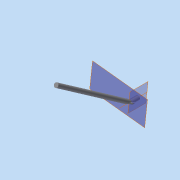
# Autodesk Inventor part: cellSTORM_lightpath
Saved by Autodesk Inventor 2019.4 (Build 234330000, 330)
## iProperties
Created: 2020-04-25
Part Number: cellSTORM_lightpath
Material: Generic
Document SubType Name: Modeling
Designer: diederichbenedict
Density: 1 g/cm^3
Appearance: Default
Mass: 3.01644 g
Surface Area: 25.0036 cm^2
Volume: 3.01644 cm^3
Author: diederichbenedict
Autodesk Inventor part; units mm, degrees
ref_plane "YZ Plane" through (0, 0, 0) normal (1, 0, 0) x (0, 1, 0)
ref_plane "XZ Plane" through (0, 0, 0) normal (0, 1, 0) x (-1, 0, 0)
ref_plane "XY Plane" through (0, 0, 0) normal (0, 0, 1) x (1, 0, 0)
ref_plane "Work Plane4" through (0, 0, 10) normal (-0.994, 0.1092, 0) x (-0.1092, -0.994, 0)
ref_plane "Work Plane3" through (-40.2485, 19.0101, 10) normal (-0.994, 0.1092, 0) x (-0.1092, -0.994, 0)
sketch "Sketch1" plane through (0, 0, 10) normal (-1, 0, 0) x (0, -1, 0)
  line L0 (0, -10) -> (0, 10)
  line L1 (0, 10) -> (-65.5322, 55.8861)
  line L2 (-7.1094, 12.5876) -> (7.1094, 7.4124)
  line L3 (-65.5322, 55.8861) -> (-90.1067, 73.0934)
  dimension "d0" = 20
  dimension "d1" = 80
  dimension "d2" = 125
  dimension "d6" = 70
  dimension "d23" = 30
  dimension "d26" = 180
  constraints: 8 end point, 1 midpoint, 1 vertical
  measures "d0" distance of L0.end L0.start
  measures "d1" distance of L1.end L0.end
  measures "d2" angle of L1 L0
  measures "d6" angle of L2 L0
  measures "d23" distance of L1.end L3.end
  measures "d26" angle of L3 L1
ref_plane "Work Plane9" through (-18.0552, 1.9841, 10) normal (0, 0, -1) x (-0.994, 0.1092, 0)
sketch "Sketch3" plane through (-18.0552, 1.9841, 10) normal (0, 0, -1) x (-0.994, 0.1092, 0)
  circle A0 centre (-18.1638, 0) radius 11.5 projected
  circle A1 centre (-18.1638, 0) radius 2.5
  point P0 (-18.1638, 0)
  dimension "d7" = 5
  constraints: 1 centre point, 1 coincident
  measures "d7" diameter of A1
sweep "Sweep1" add profiles "Sketch3" path "Sketch1" path curves L0 L1 L3 contours A1
sketch "Sketch7" plane through (0, 0, 10) normal (-1, 0, 0) x (0, -1, 0)
  line L0 (0, 10) -> (0, 10) projected
  line L1 (0, 10) -> (0, 10) projected
  line L2 (2.5, -10) -> (-2.5, -10) projected
  line L3 (0, 0) -> (0, 0) projected
  line L4 (0, 0) -> (0, 0) projected
  line L5 (2.5, -10) -> (2.5, 0.7882) projected
  line L6 (-2.5, -10) -> (-2.5, -0.7882) projected
  line L7 (-2.5, -0.7882) -> (2.8679, 0.9042) projected
  line L8 (0, -10) -> (0, 10)
  line L9 (1.4822, 5.299) -> (-7.1718, 32.746)
  line L10 (-7.1718, 32.746) -> (17.2582, 19.3562)
  line L11 (17.2582, 19.3562) -> (10.5548, 1.8291)
  line L12 (10.5548, 1.8291) -> (1.4822, 5.299)
  line L13 (-48.3403, -54.2978) -> (-48.6823, -53.3019)
  line L14 (-73.7647, -67.98) -> (-66.6763, -71.8283)
  line L15 (-66.6763, -71.8283) -> (-47.7403, -64.4229)
  line L16 (-47.7403, -64.4229) -> (-48.3403, -54.2978)
  line L17 (-55.533, -59.0685) -> (-56.5685, -56.5685) projected
  line L18 (-48.6823, -53.3019) -> (-76.2479, -64.72)
  line L19 (-76.2479, -64.72) -> (-73.7647, -67.98)
  point P0 (-65.0552, -65.9873)
  constraints: 22 end point, 2 perpendicular, 2 point on line, 1 vertical, 2 other
extrude "Extrusion4" cut sketch "Sketch7" along normal mid plane 10 contours L9 L10 L11 L12
sketch "Sketch8" plane through (0, 0, 20) normal (0, -0.9537, 0.3007) x (1, 0, 0)
  ellipse E0 centre (0, 0) end of major axis (0, 4.1067) minor radius 2.5 (2.5, 0) -> (-2.5, 0) ccw projected
  circle A0 centre (0, 0) radius 4.3056
  ellipse E1 centre (0, 0) end of major axis (0, -8.3138) minor radius 2.5 (2.0132, -4.9292) -> (2.5, 0) ccw projected
  ellipse E2 centre (0, 0) end of major axis (0, -8.3138) minor radius 2.5 (-2.5, 0) -> (-2.0132, -4.9292) ccw projected
  line L0 (-2.0132, -4.9292) -> (2.0132, -4.9292) projected
  point P0 (0, -9.5372)
  constraints: 1 centre point, 3 other
extrude "Extrusion5" add sketch "Sketch8" against normal blind 1 contours E1 A0 E2 E0 | E0 E2 A0 E1
ref_plane "Work Plane10" through (-6.4984, 57.0254, -46.7578) normal (0, -0.3827, -0.9239) x (0, -0.9239, 0.3827)
sketch "Sketch9" plane through (-6.4984, 57.0254, -46.7578) normal (0, -0.3827, -0.9239) x (0, -0.9239, 0.3827)
  ellipse E0 centre (0.4945, -6.4984) end of major axis (-6.0383, -6.4984) minor radius 2.5 projected
  circle A0 centre (0.4945, -6.4984) radius 10.9648
  point P0 (70.578, -6.4984)
  constraints: 1 centre point, 1 other
extrude "Extrusion6" add sketch "Sketch9" against normal blind 1 contours E0 | A0
ref_plane "Work Plane2" through (-1.6385, -14.9102, 10) normal (0, 0, 1) x (0.994, -0.1092, 0)
body "Solid1"
